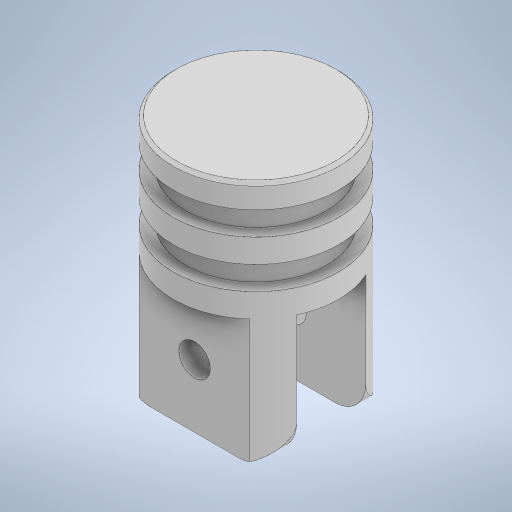
# Autodesk Inventor part: Piston Head
Saved by Autodesk Inventor 2023 (Build 270158000, 158)
## iProperties
Created: 2022-10-26
Part Number: Piston Head
Material: Generic
Document SubType Name: Modeling
Designer: tommy
Density: 1 g/cm^3
Appearance: Default
Author: tommy
Autodesk Inventor part; units mm, degrees
ref_plane "YZ Plane" through (0, 0, 0) normal (1, 0, 0) x (0, 1, 0)
ref_plane "XZ Plane" through (0, 0, 0) normal (0, 1, 0) x (-1, 0, 0)
ref_plane "XY Plane" through (0, 0, 0) normal (0, 0, 1) x (1, 0, 0)
sketch "Sketch5" plane through (0, 0, 0) normal (1, 0, 0) x (0, 1, 0)
  line L0 (15.875, -16.6688) -> (15.875, -14.2875)
  line L1 (15.875, -14.2875) -> (20.6375, -14.2875)
  line L2 (20.6375, -14.2875) -> (20.6375, -16.6688)
  line L3 (20.6375, -16.6688) -> (25.4, -16.6688)
  line L4 (25.4, -16.6688) -> (25.4, -14.2875)
  line L5 (25.4, -14.2875) -> (30.1625, -14.2875)
  line L6 (30.1625, -14.2875) -> (30.1625, -16.6688)
  line L7 (30.1625, -16.6688) -> (34.925, -16.6688)
  line L8 (34.925, -16.6688) -> (34.925, 0)
  line L9 (15.875, -16.6688) -> (11.0998, -16.6688)
  line L10 (34.925, 0) -> (11.0998, 0)
  line L11 (11.0998, -16.6688) -> (11.0998, 0)
  dimension "d15" = 2.3813
  dimension "d16" = 4.7625
  dimension "d17" = 4.7625
  dimension "d18" = 4.7625
  dimension "d19" = 4.7625
  dimension "d38" = 4.7752
  constraints: 24 end point, 4 point on line, 3 perpendicular, 2 vertical, 1 horizontal, 1 parallel
  measures "d15" distance of L0.start L0.end
  measures "d16" distance of L0.end L1.end
  measures "d17" distance of L2.end L3.end
  measures "d18" distance of L4.end L5.end
  measures "d19" distance of L6.end L7.end
  measures "d38" distance of L0.start L9.end
revolve "Revolution1" add sketch "Sketch5" angle 360 about axis through (0, 34.925, 0) along (0, -1, 0)
chamfer "Chamfer1" distance 0.635 angle 45 1 edges at (0, 34.925, 16.6688)
sketch "Sketch10" plane through (0, 11.0998, 0) normal (0, -1, 0) x (1, 0, 0)
  circle A0 centre (0, 0) radius 16.6687
  circle A1 centre (0, 0) radius 16.6687 projected
  line L0 (16.6687, 0) -> (-16.6687, 0)
  line L1 (-15.1346, -6.985) -> (15.1346, -6.985)
  line L2 (-11.1659, -12.3761) -> (11.1659, -12.3761)
  line L3 (-15.1346, 6.985) -> (15.1346, 6.985)
  line L4 (-11.1659, 12.3761) -> (11.1659, 12.3761)
  point P0 (15.1346, -6.985)
  point P1 (-15.1346, -6.985)
  point P2 (-15.1346, 6.985)
  point P3 (15.1346, 6.985)
  constraints: 10 end point, 6 point on circle, 4 symmetric about line, 2 horizontal, 1 centre point, 1 coincident
extrude "Extrusion4" add sketch "Sketch10" along normal blind 25.4 contours L3 A0 L4 | A0 L2 L1
sketch "Sketch11" plane through (-11.1659, 11.0998, 12.3761) normal (0, 0, 1) x (1, 0, 0)
  line L0 (0, 0) -> (22.3319, 0) projected
  circle A0 centre (11.1659, -12.7) radius 3.175
  line L1 (11.1659, -12.7) -> (26.3006, -12.7)
  line L2 (26.3006, 0) -> (26.3006, -25.4) projected
  line L3 (26.3006, -12.7) -> (26.3006, -19.05)
  line L4 (19.9506, -25.4) -> (11.1659, -25.4)
  line L5 (11.1659, -12.7) -> (-3.9687, -12.7)
  line L6 (-3.9687, -12.7) -> (-3.9687, -19.05)
  line L7 (2.3813, -25.4) -> (11.1659, -25.4)
  arc A1 (-3.9687, -19.05) -> (2.3813, -25.4) centre (2.3813, -19.05) ccw
  arc A2 (19.9506, -25.4) -> (26.3006, -19.05) centre (19.9506, -19.05) ccw
  line L8 (-3.9687, -12.7) -> (-7.4888, -12.7)
  line L9 (-7.4888, -12.7) -> (-7.4888, -35.2698)
  line L10 (-7.4888, -35.2698) -> (38.3229, -35.2698)
  line L11 (38.3229, -35.2698) -> (38.3229, -12.7)
  line L12 (38.3229, -12.7) -> (26.3006, -12.7)
  point P0 (11.1659, -11.0998)
  point P1 (26.3006, -19.05)
  dimension "d55" = 6.35
  dimension "d58" = 6.35
  constraints: 22 end point, 4 perpendicular, 4 point on circle, 4 tangent, 3 centre point, 3 point on line, 1 collinear, 1 equal radius, 1 horizontal
  measures "d55" diameter of A0
  measures "d58" radius of A1
extrude "Extrusion5" cut sketch "Sketch11" against normal blind 25.4 contours L1 L5 A0 | A0 L5 L1 | L12 L11 L10 L9 L8 L6 A1 L7 L4 A2 L2
body "Solid3"
